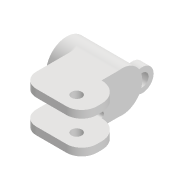
# Autodesk Inventor part: Hinge_4
Saved by Autodesk Inventor 2022 (Build 260153000, 153)
## iProperties
Created: 2022-07-08
Part Number: Hinge_4
Material: Generic
Document SubType Name: Modeling
Designer: dell
Density: 1 g/cm^3
Appearance: Default
Author: dell
Autodesk Inventor part; units mm, degrees
ref_plane "YZ Plane" through (0, 0, 0) normal (1, 0, 0) x (0, 1, 0)
ref_plane "XZ Plane" through (0, 0, 0) normal (0, 1, 0) x (-1, 0, 0)
ref_plane "XY Plane" through (0, 0, 0) normal (0, 0, 1) x (1, 0, 0)
sketch "Sketch1" plane through (0, 0, 0) normal (1, 0, 0) x (0, 1, 0)
  circle A0 centre (0, 0) radius 4.9
  circle A1 centre (0, 0) radius 6.1
  circle A2 centre (0, 0) radius 8.1
  dimension "d0" = 9.8
  dimension "d1" = 12.2
  dimension "d2" = 2
  constraints: 3 centre point, 2 coincident
  measures "d0" diameter of A0
  measures "d1" diameter of A1
  measures "d2" radial gap between concentric circles of A1 A2
extrude "Extrusion1" add sketch "Sketch1" along normal blind 20
sketch "Sketch2" plane through (20, 0, 0) normal (1, 0, 0) x (0, 0, -1)
  circle A0 centre (0, 0) radius 8.1 projected
  circle A1 centre (0, 0) radius 6.1 projected
extrude "Extrusion2" add sketch "Sketch2" along normal blind 2 contours A0 | A1
sketch "Sketch6" plane through (20, 0, 0) normal (-1, 0, 0) x (0, 0, 1)
  circle A0 centre (0, 0) radius 4.9 projected
  circle A1 centre (0, 0) radius 6.1 projected
sketch "Sketch11" plane through (22, 0, 0) normal (1, 0, 0) x (0, 0, -1)
  line L0 (-24, 8) -> (0, 8)
  line L1 (0, 8) -> (0, 5)
  line L2 (0, 5) -> (-24, 5)
  line L3 (-24, 5) -> (-24, 8)
  point P0 (0, 0)
  dimension "d57" = 5
  dimension "d58" = 3
  dimension "d60" = 24
  constraints: 8 end point, 2 parallel, 1 horizontal, 1 perpendicular, 1 point on line
  measures "d57" distance from line of point (0, 0) L2
  measures "d58" distance between parallel lines of L2 L0
  measures "d60" distance between parallel lines of L1 L3
extrude "Extrusion9" add sketch "Sketch11" along normal blind 8 and the other way blind 16
sketch "Sketch12" plane through (22, 8, 1.2689) normal (0, 1, 0) x (1, 0, 0)
  circle A0 centre (0, -16.7311) radius 2.05
  line L0 (8, 1.2689) -> (8, -22.7311) projected
  line L1 (-16, -22.7311) -> (8, -22.7311) projected
  line L2 (8, -22.7311) -> (8, 1.2689) projected
  point P0 (-22, 1.2689)
  dimension "d63" = 4.1
  dimension "d64" = 8
  dimension "d65" = 6
  constraints: 1 centre point
  measures "d63" diameter of A0
  measures "d64" distance from line of L0 A0.centre
  measures "d65" distance from line of L1 A0.centre
extrude "Extrusion10" cut sketch "Sketch12" against normal blind 32
fillet "Fillet5" radius 6 3 edges at (6, 6.5, 24) (30, 6.5, 24) (14, 8, 1.2689)
fillet "Fillet6" radius 1 2 edges at (14, 5, 6.3726) (6, 7.06, 3.9708)
mirror "Mirror1" about plane through (0, 0, 0) normal (0, 1, 0) of "Extrusion9", "Extrusion10", "Fillet5", "Fillet6"
sketch "Sketch14" plane through (22, 0, 0) normal (1, 0, 0) x (0, 0, -1)
  line L0 (8.1, -8.1) -> (-8.1, -8.1)
  line L1 (-8.1, -8.1) -> (-8.1, 8.1)
  line L2 (-8.1, 8.1) -> (8.1, 8.1)
  line L3 (8.1, 8.1) -> (8.1, -8.1)
  line L4 (8.1, -8.1) -> (-8.1, 8.1) construction
  line L5 (-8.1, -8.1) -> (8.1, 8.1) construction
  point P0 (0, 0)
  dimension "d70" = 16.2
  dimension "d71" = 16.2
  constraints: 12 end point, 2 midpoint, 2 parallel, 1 horizontal, 1 perpendicular
  measures "d70" distance of L1.end L2.end
  measures "d71" distance of L0.end L1.end
extrude "Extrusion11" cut sketch "Sketch14" along normal blind 100
extrude "Extrusion12" cut sketch "Sketch6" along normal blind 100
fillet "Fillet7" radius 8 2 edges at (30, 6.5, 8.1) (30, -6.5, 8.1)
sketch "Sketch15" plane through (22, 0, 0) normal (1, 0, 0) x (0, 0, -1)
  arc A0 (-0.963, -8.0426) -> (-0.963, 8.0426) centre (0, 0) ccw projected
  circle A1 centre (0, 0) radius 8.1 projected
  circle A2 centre (8.1, 0) radius 2.5
  circle A3 centre (8.1, 0) radius 4.5
  point P0 (6.85, 4.3229)
  point P1 (7.7142, 2.4701)
  point P2 (7.7142, -2.4701)
  point P3 (6.85, -4.3229)
  dimension "d79" = 5
  dimension "d80" = 2
  constraints: 2 centre point, 2 point on circle
  measures "d79" diameter of A2
  measures "d80" radial gap between concentric circles of A2 A3
extrude "Extrusion13" add sketch "Sketch15" against normal blind 4 contours A0 A2 A3 picked at (11.8933, -0.3442)
body "Solid1"
